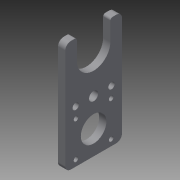
# Autodesk Inventor part: motor mount
Saved by Autodesk Inventor 2015 SP1 (Build 190203100, 203)
## iProperties
Created: 2016-07-07
Part Number: motor mount
Material: Generic
Document SubType Name: Modeling
Designer: lustinga
Density: 1 g/cm^3
Appearance: Default
Mass: 10.8386 g
Surface Area: 85.0658 cm^2
Volume: 10.8386 cm^3
Author: lustinga
Autodesk Inventor part; units mm, degrees
ref_plane "YZ Plane" through (0, 0, 0) normal (1, 0, 0) x (0, 1, 0)
ref_plane "XZ Plane" through (0, 0, 0) normal (0, 1, 0) x (-1, 0, 0)
ref_plane "XY Plane" through (0, 0, 0) normal (0, 0, 1) x (1, 0, 0)
sketch "Sketch1" plane through (0, 0, 0) normal (1, 0, 0) x (0, 1, 0)
  circle A0 centre (31.2856, 22.5008) radius 2
  circle A1 centre (31.2537, -8.4991) radius 2
  circle A2 centre (0.2856, 22.5008) radius 2
  circle A3 centre (0.2537, -8.4991) radius 2
  arc A4 (1.0356, 66.0111) -> (30.5356, 66.0111) centre (15.7856, 66.0009) ccw
  line L0 (30.5356, 66.0111) -> (30.5356, 82.0008)
  line L1 (-4.2145, -13.9991) -> (35.7855, -13.9992)
  line L2 (40.7858, 79.0008) -> (40.7855, -8.9992)
  circle A5 centre (15.7856, 32.0009) radius 4
  circle A6 centre (15.7856, 7.0009) radius 11.25
  line L3 (-9.2144, 79.0009) -> (-9.2145, -8.9991)
  line L4 (1.0356, 66.0111) -> (1.0356, 82.0009)
  line L5 (-4.2144, 84.0009) -> (-0.9644, 84.0009)
  line L6 (32.5356, 84.0008) -> (35.7858, 84.0008)
  circle A7 centre (0.0356, 32.0009) radius 2.8
  circle A8 centre (31.5356, 32.0009) radius 2.8
  line L7 (15.7856, 32.0009) -> (15.7856, 45.0825) construction
  arc A9 (-9.2145, -8.9991) -> (-4.2145, -13.9991) centre (-4.2145, -8.9991) ccw
  arc A10 (35.7855, -13.9992) -> (40.7855, -8.9992) centre (35.7855, -8.9992) ccw
  arc A11 (40.7858, 79.0008) -> (35.7858, 84.0008) centre (35.7858, 79.0008) ccw
  arc A12 (-4.2144, 84.0009) -> (-9.2144, 79.0009) centre (-4.2144, 79.0009) ccw
  arc A13 (1.0356, 82.0009) -> (-0.9644, 84.0009) centre (-0.9644, 82.0009) ccw
  arc A14 (32.5356, 84.0008) -> (30.5356, 82.0008) centre (32.5356, 82.0008) ccw
  point P0 (-9.2144, 84.0009)
  point P1 (30.5356, 84.0008)
  point P2 (-9.2145, -13.9991)
  point P3 (40.7855, -13.9992)
  point P4 (40.7859, 84.0008)
  point P5 (1.0356, 84.0009)
  dimension "d5" = 31
  dimension "d6" = 31
  dimension "d8" = 31
  dimension "d21" = 29.5
  dimension "d44" = 8
  dimension "d46" = 80
  dimension "d47" = 22.5
  dimension "d49" = 98
  dimension "d56" = 50
  dimension "d57" = 25
  dimension "d58" = 15.5
  dimension "d61" = 21
  dimension "d62" = 46
  dimension "d63" = 5.6
  dimension "d64" = 5.6
  dimension "d65" = 15.75
  dimension "d66" = 15.75
  dimension "d67" = 25
  dimension "d70" = 31
  dimension "d71" = 15.5
  dimension "d72" = 15.5
  dimension "d73" = 4
  dimension "d74" = 18
  dimension "d75" = 5
  dimension "d76" = 5
  dimension "d77" = 2
  constraints: 16 end point, 15 centre point, 14 point on circle, 12 point on line, 12 tangent, 6 equal radius, 3 vertical, 2 equal length, 2 vertical alignment, 1 coincident, 1 horizontal, 1 other
  measures "d5" distance of A0.centre A2.centre
  measures "d6" distance of A1.centre A0.centre
  measures "d8" distance of A2.centre A3.centre
  measures "d21" diameter of A4
  measures "d44" diameter of A5
  measures "d46" distance from line of L1 A4.centre
  measures "d47" diameter of A6
  measures "d49" distance of point (-9.215, -13.999) point (-9.214, 84.001)
  measures "d56" distance of point (-9.215, -13.999) point (40.785, -13.999)
  measures "d57" distance from line of L3 A4.centre
  measures "d58" horizontal distance of A2.centre A6.centre
  measures "d61" distance from line of L1 A6.centre
  measures "d62" distance from line of L1 L7.start
  measures "d63" diameter of A7
  measures "d64" diameter of A8
  measures "d65" distance of L7.start A8.centre
  measures "d66" distance of point (15.786, 32.001) A7.centre
  measures "d67" distance from line of L2 A6.centre
  measures "d70" distance of A1.centre A3.centre
  measures "d71" vertical distance of A6.centre A3.centre
  measures "d72" vertical distance of A6.centre A1.centre
  measures "d73" diameter of A3
  measures "d74" distance from line of L5 A4.centre
  measures "d75" radius of A9
  measures "d76" radius of A11
  measures "d77" radius of A13
extrude "Extrusion2" add sketch "Sketch1" along normal blind 6.35
body "Solid2"
